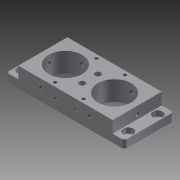
# Autodesk Inventor part: 13_0204_049
Saved by Autodesk Inventor 2012 SP1 (Build 160190100, 190)
## iProperties
Created: 2013-04-11
Part Number: 13_0204_049
Material: Default
Document SubType Name: Modeling
Designer: vogel
Density: 1 g/cm^3
Author: vogel
Autodesk Inventor part; units mm, degrees
note: some values were not read from the file. Chosen so that the rebuilt part matches the saved one: direction of "Bohrung3"; direction of "Bohrung4".
ref_plane "YZ Plane" through (0, 0, 0) normal (1, 0, 0) x (0, 1, 0)
ref_plane "XZ Plane" through (0, 0, 0) normal (0, 1, 0) x (-1, 0, 0)
ref_plane "XY Plane" through (0, 0, 0) normal (0, 0, 1) x (1, 0, 0)
sketch "Skizze1" plane through (0, 0, 0) normal (0, 0, 1) x (1, 0, 0)
  line L0 (-60, 25) -> (60, 25)
  line L1 (60, 25) -> (60, -25)
  line L2 (60, -25) -> (-60, -25)
  line L3 (-60, -25) -> (-60, 25)
  line L4 (-84, 0) -> (84, 0) projected
  line L5 (0, -35) -> (0, 35) projected
  circle A0 centre (-25, 0) radius 17
  circle A1 centre (25, 0) radius 17
  point P0 (0, 0)
  dimension "d0" = 50
  dimension "d1" = 34
  dimension "d2" = 50
  dimension "d3" = 120
  constraints: 8 end point, 2 centre point, 2 coincident, 2 parallel, 2 point on line, 1 equal radius, 1 horizontal, 1 perpendicular, 1 symmetric about line, 2 other
  measures "d0" distance of point (25, 0) point (-25, 0)
  measures "d1" diameter of A0
  measures "d2" distance of L2.end L0.start
  measures "d3" distance of L1.end L2.end
extrude "Extrusion1" add sketch "Skizze1" along normal blind 20 contours L0 L5 L4 A0 L3 | L0 L1 L4 A1 L5 | L4 A0 L5 L2 L3 | L4 A1 L1 L2 L5
sketch "Skizze2" plane through (0, 0, 20) normal (0, 0, 1) x (1, 0, 0)
  line L0 (-84, 0) -> (84, 0) projected
  line L1 (0, -35) -> (0, 35) projected
  point P0 (0, 0)
  point P1 (0, 8)
  point P2 (0, -8)
  dimension "d6" = 16
  constraints: 2 point on line, 1 symmetric about line
  measures "d6" distance of point (0, -8) point (0, 8)
hole "Bohrung1" at (0, 8, 20) at (0, -8, 20) direction (0, 0, -1) diameter 6 end through all
sketch "Skizze3" plane through (-60, -25, 0) normal (0, -1, 0) x (1, 0, 0)
  line L0 (120, 20) -> (0, 20) projected
  line L1 (0, 0) -> (0, 20) projected
  line L2 (120, 0) -> (0, 0) projected
  line L3 (120, 0) -> (120, 20) projected
  line L4 (0, 8) -> (12, 8)
  line L5 (12, 8) -> (12, 20)
  line L6 (12, 20) -> (0, 20)
  line L7 (0, 20) -> (0, 8)
  line L8 (120, 8) -> (108, 8)
  line L9 (108, 8) -> (108, 20)
  line L10 (108, 20) -> (120, 20)
  line L11 (120, 20) -> (120, 8)
  line L12 (-24, 0) -> (144, 0) projected
  line L13 (60, -4) -> (60, 24) projected
  point P0 (60, 0)
  dimension "d14" = 12
  dimension "d15" = 8
  constraints: 16 end point, 4 parallel, 4 point on line, 2 horizontal, 2 perpendicular, 1 collinear, 1 other
  measures "d14" distance of L5.end L6.end
  measures "d15" distance between parallel lines of L4 L2
extrude "Extrusion2" cut sketch "Skizze3" against normal through all contours L3 L8 L9 L0 | L5 L4 L1 L0
sketch "Skizze4" plane through (-60, -25, 0) normal (0, -1, 0) x (1, 0, 0)
  line L0 (108, 8) -> (108, 20) projected
  line L1 (108, 20) -> (12, 20) projected
  line L2 (12, 20) -> (12, 8) projected
  line L3 (-24, 0) -> (144, 0) projected
  line L4 (60, -4) -> (60, 24) projected
  line L5 (12, 12) -> (108, 12)
  point P0 (60, 0)
  point P1 (35, 12)
  point P2 (85, 12)
  dimension "d18" = 8
  dimension "d19" = 50
  constraints: 4 point on line, 2 end point, 1 perpendicular, 1 symmetric about line
  measures "d18" distance between parallel lines of L1 L5
  measures "d19" distance of point (85, 12) point (35, 12)
hole "Bohrung2" at (-25, -25, 12) at (25, -25, 12) direction (0, 1, 0) diameter 4.134 end through all thread size "M5x0.8" class "6H" standard "ISO Metric profile"
sketch "Skizze5" plane through (-48, -25, 8) normal (-1, 0, 0) x (0, 0, 1)
  line L0 (12, 50) -> (12, 0) projected
  line L1 (-8, -10) -> (-8, 60) projected
  line L2 (-12, 25) -> (16, 25) projected
  point P0 (-8, 25)
  point P1 (4, 25)
  dimension "d27" = 8
  constraints: 1 point on line
  measures "d27" distance from line of point (4, 25) L0
hole "Bohrung3" at (-48, 0, 12) direction (1, 0, 0) diameter 4.134 end up to surface thread size "M5x0.8" class "6H" standard "ISO Metric profile"
sketch "Skizze6" plane through (48, -25, 20) normal (1, 0, 0) x (0, 0, -1)
  line L0 (0, 0) -> (0, 50) projected
  line L1 (20, -10) -> (20, 60) projected
  line L2 (24, 25) -> (-4, 25) projected
  point P0 (20, 25)
  point P1 (8, 25)
  dimension "d35" = 8
  constraints: 1 point on line
  measures "d35" distance from line of point (8, 25) L0
hole "Bohrung4" at (48, 0, 12) direction (-1, 0, 0) diameter 4.134 end up to surface thread size "M5x0.8" class "6H" standard "ISO Metric profile"
sketch "Skizze7" plane through (0, 0, 20) normal (0, 0, 1) x (1, 0, 0)
  circle A0 centre (-14.5, 21) radius 2.25 projected
  circle A1 centre (14.5, 21) radius 2.25 projected
  line L0 (-48, 25) -> (-48, -25) projected
  line L1 (48, -25) -> (-48, -25) projected
  line L2 (48, -25) -> (48, 25) projected
  line L3 (-48, 25) -> (48, 25) projected
  circle A2 centre (0, -8) radius 3 projected
  circle A3 centre (0, 8) radius 3 projected
  circle A4 centre (25, 0) radius 17 projected
  circle A5 centre (-25, 0) radius 17 projected
  circle A6 centre (14.5, -21) radius 2.25 projected
  circle A7 centre (-14.5, -21) radius 2.25 projected
  point P0 (0, 0)
  constraints: 4 coincident
hole "Bohrung5" at (-14.5, -21, 20) at (14.5, -21, 20) at (14.5, 21, 20) at (-14.5, 21, 20) direction (0, 0, -1) diameter 3.242 depth 10 tip angle 118 thread size "M4x0.7" class "6H" standard "ISO Metric profile"
sketch "Skizze8" plane through (0, 0, 0) normal (0, 0, -1) x (-1, 0, 0)
  circle A0 centre (0, -8) radius 3 projected
  circle A1 centre (0, 8) radius 3 projected
  circle A2 centre (0, 8) radius 4.5
  circle A3 centre (0, -8) radius 4.5
  point P0 (0, 0)
  dimension "d50" = 9
  constraints: 2 centre point, 2 coincident, 1 equal radius
  measures "d50" diameter of A2
extrude "Extrusion3" cut sketch "Skizze8" against normal blind 2
sketch "Skizze9" plane through (48, -25, 8) normal (0, 0, 1) x (1, 0, 0)
  line L0 (0, 50) -> (12, 50) projected
  line L1 (12, 0) -> (0, 0) projected
  line L2 (12, 50) -> (12, 0) projected
  line L3 (6, 50) -> (6, 0)
  line L4 (-108, 50) -> (-96, 50) projected
  line L5 (-108, 0) -> (-108, 50) projected
  line L6 (-96, 0) -> (-108, 0) projected
  line L7 (-96, 0) -> (-96, 50) projected
  line L8 (-102, 50) -> (-102, 0)
  line L9 (-108, 25) -> (12, 25)
  point P0 (-48, 25)
  point P1 (-102, 40)
  point P2 (-102, 10)
  point P3 (6, 40)
  point P4 (6, 10)
  dimension "d53" = 30
  constraints: 6 end point, 6 midpoint, 4 point on line, 2 symmetric about line, 1 horizontal alignment
  measures "d53" distance of point (-102, 10) point (-102, 40)
hole "Bohrung6" at (-54, 15, 8) at (-54, -15, 8) at (54, 15, 8) at (54, -15, 8) direction (0, 0, -1) diameter 5.5 end through all counterbore diameter 10 counterbore depth 5.5
chamfer "Fase1" distance 2 angle 45 4 edges at (60, 25, 4) (60, -25, 4) (-60, 25, 4) (-60, -25, 4)
sketch "Skizze11" plane through (-48, -25, 8) normal (-1, 0, 0) x (0, 0, 1)
  line L0 (0, 50) -> (12, 50) projected
  line L1 (0, 0) -> (0, 50) projected
  line L2 (12, 50) -> (12, 0) projected
  line L3 (5, 51.1026) -> (5, 11.0542)
  line L4 (12, 25) -> (9.2685, 25)
  point P0 (-8, 25)
  point P1 (5, 45)
  point P2 (5, 5)
  dimension "d71" = 5
  dimension "d72" = 5
  constraints: 4 end point, 2 point on line, 1 midpoint, 1 parallel, 1 perpendicular, 1 symmetric about line
  measures "d71" distance from line of L0 point (5, 45)
  measures "d72" distance between parallel lines of L1 L3
hole "Bohrung8" at (-48, 20, 13) at (-48, -20, 13) direction (1, 0, 0) diameter 2.459 depth 10 tip angle 118 thread size "M3x0.5" class "6H" standard "ISO Metric profile"
sketch "Skizze12" plane through (-48, -25, 20) normal (0, -1, 0) x (1, 0, 0)
  line L0 (106, -20) -> (-10, -20) projected
  line L1 (96, 0) -> (0, 0) projected
  line L2 (0, -12) -> (-10, -12) projected
  line L3 (35.6086, -10) -> (62.3206, -10)
  line L4 (48, -20) -> (48, 0)
  point P0 (38, -10)
  point P1 (58, -10)
  dimension "d80" = 10
  dimension "d81" = 20
  constraints: 4 end point, 2 point on line, 1 midpoint, 1 parallel, 1 symmetric about line
  measures "d80" distance between parallel lines of L3 L0
  measures "d81" distance of point (58, -10) point (38, -10)
hole "Bohrung9" at (-10, -25, 10) at (10, -25, 10) direction (0, 1, 0) diameter 3.242 depth 10 tip angle 118 thread size "M4x0.7" class "6H" standard "ISO Metric profile"
